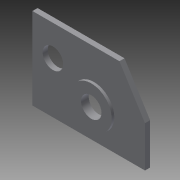
# Autodesk Inventor part: 5-2
Saved by Autodesk Inventor 2015 SP2 (Build 190223200, 223)
## iProperties
Created: 2015-09-23
Part Number: 5-2
Material: Generic
Document SubType Name: Modeling
Designer: Brandon
Density: 1 g/cm^3
Appearance: Default
Author: Brandon
Autodesk Inventor part; units mm, degrees
ref_plane "YZ Plane" through (0, 0, 0) normal (1, 0, 0) x (0, 1, 0)
ref_plane "XZ Plane" through (0, 0, 0) normal (0, 1, 0) x (-1, 0, 0)
ref_plane "XY Plane" through (0, 0, 0) normal (0, 0, 1) x (1, 0, 0)
sketch "Sketch1" plane through (0, 0, 0) normal (0, 0, 1) x (1, 0, 0)
  circle A0 centre (0, 0) radius 12.7
  circle A1 centre (0, 0) radius 25.4
  line L0 (-76.2, -38.1) -> (63.5, -38.1)
  line L1 (63.5, -38.1) -> (63.5, 12.7)
  line L2 (31.75, 63.5) -> (-76.2, 63.5)
  line L3 (-76.2, 63.5) -> (-76.2, -38.1)
  line L4 (-76.2, 63.5) -> (31.75, 63.5)
  line L5 (63.5, -38.1) -> (63.5, 12.7)
  line L6 (63.5, 12.7) -> (31.75, 63.5)
  circle A2 centre (-50.8, 25.4) radius 12.7
  dimension "d0" = 25.4
  dimension "d1" = 50.8
  dimension "d4" = 76.2
  dimension "d5" = 38.1
  dimension "d6" = 101.6
  dimension "d7" = 139.7
  dimension "d8" = 107.95
  dimension "d9" = 50.8
  dimension "d10" = 25.4
  dimension "d11" = 25.4
  dimension "d12" = 63.5
  constraints: 14 end point, 3 centre point, 2 coincident, 2 parallel, 1 horizontal, 1 perpendicular
  measures "d0" diameter of A0
  measures "d1" diameter of A1
  measures "d4" distance from line of L3 point (0, 0)
  measures "d5" vertical distance of L0.end point (0, 0)
  measures "d6" distance of L2.end L0.start
  measures "d7" distance of L0.start L0.end
  measures "d8" distance of L2.start L2.end
  measures "d9" distance of L1.end L0.end
  measures "d10" diameter of A2
  measures "d11" horizontal distance of L2.end A2.centre
  measures "d12" vertical distance of L0.start A2.centre
extrude "Extrusion1" add sketch "Sketch1" along normal blind 6.35 contours A1 | L3 L2 L6 L1 L0
sketch "Sketch2" plane through (0, 0, 6.35) normal (0, 0, 1) x (1, 0, 0)
  circle A0 centre (0, 0) radius 12.7
  circle A1 centre (0, 0) radius 25.4
  dimension "d15" = 25.4
  dimension "d16" = 50.8
  constraints: 2 centre point, 2 coincident
  measures "d15" diameter of A0
  measures "d16" diameter of A1
extrude "Extrusion2" add sketch "Sketch2" along normal blind 3.175
body "Solid1"
